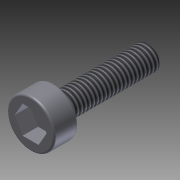
# Autodesk Inventor part: 10 32 bolt 0.75
Saved by Autodesk Inventor 2012 (Build 160160000, 160)
## iProperties
Created: 2013-08-29
Part Number: 10 32 bolt 0.75
Material: Default
Document SubType Name: Modeling
Designer: Bryce
Density: 1 g/cm^3
Author: Bryce
Autodesk Inventor part; units mm, degrees
ref_plane "YZ Plane" through (0, 0, 0) normal (1, 0, 0) x (0, 1, 0)
ref_plane "XZ Plane" through (0, 0, 0) normal (0, 1, 0) x (-1, 0, 0)
ref_plane "XY Plane" through (0, 0, 0) normal (0, 0, 1) x (1, 0, 0)
sketch "Sketch1" plane through (0, 0, 0) normal (0, 0, 1) x (1, 0, 0)
  circle A0 centre (0, 0) radius 2.413
  circle A1 centre (0, 0) radius 4.7625
  line L0 (1.604, 2.7781) -> (3.2079, 0)
  line L1 (3.2079, 0) -> (1.604, -2.7781)
  line L2 (1.604, -2.7781) -> (-1.604, -2.7781)
  line L3 (-1.604, -2.7781) -> (-3.2079, 0)
  line L4 (-3.2079, 0) -> (-1.604, 2.7781)
  line L5 (-1.604, 2.7781) -> (1.604, 2.7781)
  dimension "d0" = 4.826
  dimension "d1" = 9.525
  dimension "d2" = 5.5563
  constraints: 12 end point, 3 coincident, 2 centre point, 1 horizontal, 13 other
  measures "d0" diameter of A0
  measures "d1" diameter of A1
  measures "d2" distance between parallel lines of L2 L5
extrude "Extrusion1" add sketch "Sketch1" against normal blind 19.05 contours A0
extrude "Extrusion2" add sketch "Sketch1" along normal blind 4.7625 contours A1
extrude "Extrusion3" add sketch "Sketch1" along normal blind 1.651 contours A0 | L0 L1 L2 L3 L4 L5
thread "Thread1" size "10-32 UNF" class "2A" standard "ANSI Unified Screw Threads" full length
chamfer "Chamfer1" distance 0.3969 angle 45 1 edges at (-2.413, 0, -19.05)
fillet "Fillet1" radius 0.3969 2 edges at (-4.7625, 0, 0) (-4.7625, 0, 4.7625)
body "Solid1"
